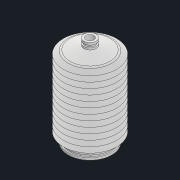
# Autodesk Inventor part: Boot
Saved by Autodesk Inventor 2021 (Build 250183000, 183)
## iProperties
Created: 2020-10-22
Part Number: Boot
Material: Generic
Document SubType Name: Modeling
Designer: Tang Kang Ning
Mass: 84.9799 g
Surface Area: 1568.76 cm^2
Volume: 84.9799 cm^3
Density: 1 g/cm^3
Appearance: Default
Author: Tang Kang Ning
Autodesk Inventor part; units mm, degrees
ref_plane "YZ Plane" through (0, 0, 0) normal (1, 0, 0) x (0, 1, 0)
ref_plane "XZ Plane" through (0, 0, 0) normal (0, 1, 0) x (-1, 0, 0)
ref_plane "XY Plane" through (0, 0, 0) normal (0, 0, 1) x (1, 0, 0)
sketch "Sketch1" plane through (0, 0, 0) normal (0, 0, 1) x (1, 0, 0)
  line L0 (-37, 65.25) -> (37, 65.25) projected
  line L1 (-37, 53.25) -> (37, 53.25) projected
  line L2 (35, 65.25) -> (35, 53.25)
  line L3 (-9, 215.6144) -> (9, 215.6144) projected
  line L4 (7, 215.6144) -> (7, 203.6144)
  line L5 (-9, 203.6144) -> (9, 203.6144) projected
  line L6 (7, 215.6144) -> (7, 203.6144)
  line L7 (9, 203.6144) -> (7, 203.6144)
  line L8 (7, 215.6144) -> (11, 215.6144)
  line L9 (35, 53.25) -> (39, 53.25)
  line L10 (39, 53.25) -> (39, 57.25)
  line L11 (39, 57.25) -> (37, 57.25)
  line L12 (37, 57.25) -> (37, 61.25)
  line L13 (37, 61.25) -> (39, 61.25)
  line L14 (39, 61.25) -> (39, 65.25)
  line L15 (39, 65.25) -> (37, 65.25) construction
  line L16 (11, 215.6144) -> (11, 211.6144)
  line L17 (11, 211.6144) -> (9, 211.6144)
  line L18 (9, 211.6144) -> (9, 207.6144)
  line L19 (9, 207.6144) -> (11, 207.6144)
  line L20 (11, 207.6144) -> (11, 203.6144)
  line L21 (7, 215.6144) -> (7, 203.6144)
  line L22 (39, 65.25) -> (47.6603, 70.25)
  line L23 (37, 65.25) -> (45.6603, 70.25)
  line L24 (37, 65.25) -> (37, 83.6946) construction
  line L25 (45.6603, 70.25) -> (37, 70.25) construction
  line L26 (45.6603, 70.25) -> (37, 75.25)
  line L27 (47.6603, 70.25) -> (39, 75.25)
  line L28 (35.6266, 196.7039) -> (11, 204.0606)
  line L29 (37, 195.25) -> (9, 203.6144)
  line L30 (37, 75.25) -> (46.1526, 75.25) construction
  line L31 (45.6603, 80.25) -> (37, 85.25)
  line L32 (47.6603, 80.25) -> (39, 85.25)
  line L33 (39, 75.25) -> (47.6603, 80.25)
  line L34 (37, 75.25) -> (45.6603, 80.25)
  line L35 (45.6603, 90.25) -> (37, 95.25)
  line L36 (47.6603, 90.25) -> (39, 95.25)
  line L37 (39, 85.25) -> (47.6603, 90.25)
  line L38 (37, 85.25) -> (45.6603, 90.25)
  line L39 (45.6603, 100.25) -> (37, 105.25)
  line L40 (47.6603, 100.25) -> (39, 105.25)
  line L41 (39, 95.25) -> (47.6603, 100.25)
  line L42 (37, 95.25) -> (45.6603, 100.25)
  line L43 (45.6603, 110.25) -> (37, 115.25)
  line L44 (47.6603, 110.25) -> (39, 115.25)
  line L45 (39, 105.25) -> (47.6603, 110.25)
  line L46 (37, 105.25) -> (45.6603, 110.25)
  line L47 (45.6603, 120.25) -> (37, 125.25)
  line L48 (47.6603, 120.25) -> (39, 125.25)
  line L49 (39, 115.25) -> (47.6603, 120.25)
  line L50 (37, 115.25) -> (45.6603, 120.25)
  line L51 (45.6603, 130.25) -> (37, 135.25)
  line L52 (47.6603, 130.25) -> (39, 135.25)
  line L53 (39, 125.25) -> (47.6603, 130.25)
  line L54 (37, 125.25) -> (45.6603, 130.25)
  line L55 (45.6603, 140.25) -> (37, 145.25)
  line L56 (47.6603, 140.25) -> (39, 145.25)
  line L57 (39, 135.25) -> (47.6603, 140.25)
  line L58 (37, 135.25) -> (45.6603, 140.25)
  line L59 (45.6603, 150.25) -> (37, 155.25)
  line L60 (47.6603, 150.25) -> (39, 155.25)
  line L61 (39, 145.25) -> (47.6603, 150.25)
  line L62 (37, 145.25) -> (45.6603, 150.25)
  line L63 (45.6603, 160.25) -> (37, 165.25)
  line L64 (47.6603, 160.25) -> (39, 165.25)
  line L65 (39, 155.25) -> (47.6603, 160.25)
  line L66 (37, 155.25) -> (45.6603, 160.25)
  line L67 (45.6603, 170.25) -> (37, 175.25)
  line L68 (47.6603, 170.25) -> (39, 175.25)
  line L69 (39, 165.25) -> (47.6603, 170.25)
  line L70 (37, 165.25) -> (45.6603, 170.25)
  line L71 (45.6603, 180.25) -> (37, 185.25)
  line L72 (47.6603, 180.25) -> (39, 185.25)
  line L73 (39, 175.25) -> (47.6603, 180.25)
  line L74 (37, 175.25) -> (45.6603, 180.25)
  line L75 (45.6603, 190.25) -> (37, 195.25)
  line L76 (47.6603, 190.25) -> (39, 195.25)
  line L77 (39, 185.25) -> (47.6603, 190.25)
  line L78 (37, 185.25) -> (45.6603, 190.25)
  arc A0 (39, 195.25) -> (35.6266, 196.7039) centre (31.1099, 181.5839) ccw
  line L79 (0, -43.1229) -> (0, 258.7373) projected
  point P0 (0, 0)
  dimension "d0" = 4
  dimension "d1" = 12
  dimension "d2" = 4
  dimension "d3" = 2
  dimension "d4" = 2
  dimension "d5" = 4
  dimension "d6" = 4
  dimension "d7" = 2
  dimension "d8" = 2
  dimension "d9" = 150.3644
  dimension "d10" = 150.3644
  dimension "d12" = 120
  dimension "d13" = 1
  dimension "d17" = 10
  dimension "d18" = 10
  dimension "d28" = 10
  dimension "d33" = 1
  dimension "d34" = 12
  dimension "d35" = 4
  constraints: 150 end point, 13 perpendicular, 9 point on line, 5 vertical, 3 parallel, 2 horizontal, 2 point on circle, 2 tangent, 1 centre point, 1 coincident, 1 collinear, 1 equal length, 124 other
  measures "d0" distance between parallel lines of L15 L13
  measures "d1" distance of L2.start L2.end
  measures "d2" distance between parallel lines of L9 L11
  measures "d3" distance between parallel lines of L12 L14
  measures "d4" distance between parallel lines of L2 L12
  measures "d5" distance of L8.end L16.end
  measures "d6" distance of L19.end L20.end
  measures "d7" distance between parallel lines of L4 L18
  measures "d8" distance between parallel lines of L18 L20
  measures "d9" distance between parallel lines of L1 L5
  measures "d10" distance between parallel lines of L1 L7
  measures "d12" angle of L14 L22
  measures "d13" distance between parallel lines of L22 L23
  measures "d17" distance of L14.end L22.end
  measures "d18" distance of L0.end L26.end
  measures "d28" distance of L23.end L31.start
  measures "d33" distance between parallel lines of L28 L29
  measures "d34" distance of L4.start L4.end
  measures "d35" distance between parallel lines of L7 L19
revolve "Revolution1" add sketch "Sketch1" angle 360 about axis through (0, -10, 0) along (0, 1, 0) contours L0 L23 L26 L34 L31 L38 L35 L42 L39 L46 L43 L50 L47 L54 L51 L58 L55 L62 L59 L66 L63 L70 L67 L74 L71 L78 L75 L29 L5 L4 L3 L8 L16 L17 L18 L19 L20 L28 A0 L76 L77 L72 L73 L68 L69 L64 L65 L60 L61 L56 L57 L52 L53 L48 L49 L44 L45 L40 L41 L36 L37 L32 L33 L27 L22 L14 L13 L12 L11 L10 L9 L1 L2
equation "\"d0\" = 0.333333 * d1"
equation "\"d2\" = d0"
equation "\"d5\" = d0"
equation "\"d6\" = d0"
equation "\"d10\" = d9"
equation "\"d28\" = d18"
equation "\"d33\" = d13"
body "Solid1"
